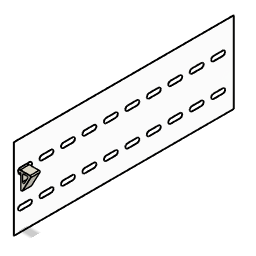
250711 TnH climate chamber wall shelf mount (Autodesk Fusion 360 design; units mm, degrees)
Autodesk Fusion 360 part; units mm, degrees
sketch "Sketch1" plane through (0, 0, 0) normal (1, 0, 0) x (0, 0, -1)
  line L0 (0, 0) -> (130.389561, 0) construction
  line L1 (0, 5) -> (20, 5)
  line L2 (0, -5) -> (20, -5)
  arc A0 (20, -5) -> (20, 5) centre (20, 0) ccw
  arc A1 (0, 5) -> (0, -5) centre (0, 0) ccw
  dimension "d1" = 10
  dimension "d2" = 10
  dimension "d3" = 20
  constraint coincident L0.start A1.centre
  constraint horizontal L0
  constraint coincident L0 A0.centre
  constraint tangent L1 A0
  constraint parallel L0 L1
  constraint tangent L2 A0
  constraint parallel L0 L2
  measures "d1" diameter of A0
  measures "d2" diameter of A1
  measures "d3" distance of L0.start A0.centre
extrude "Extrude1" add sketch "Sketch1" along normal blind 5 contours L1 L2 A0 A1 picked at (13.333333, -1.666667) makes body 1
pattern_linear "R-Pattern1" count 2 spacing 70 along (0, 1, 0) count 10 spacing 46 along (0, 0, -1) of bodies 1 makes body 2 at (0, 68.333333, -13.333333) makes body 3 at (0, -1.666667, -59.333333) makes body 4 at (0, 68.333333, -59.333333) makes body 5 at (0, -1.666667, -105.333333) makes body 6 at (0, 68.333333, -105.333333) makes body 7 at (0, -1.666667, -151.333333) makes body 8 at (0, 68.333333, -144.666667) makes body 9 at (0, -1.666667, -197.333333) makes body 10 at (0, 68.333333, -190.666667) makes body 11 at (0, -1.666667, -243.333333) makes body 12 at (0, 68.333333, -236.666667) makes body 13 at (0, -1.666667, -289.333333) makes body 14 at (0, 68.333333, -282.666667) makes body 15 at (0, -1.666667, -335.333333) makes body 16 at (0, 68.333333, -328.666667) makes body 17 at (0, -1.666667, -381.333333) makes body 18 at (0, 68.333333, -374.666667) makes body 19 at (0, -1.666667, -427.333333) makes body 20 at (0, 68.333333, -420.666667)
sketch "Sketch2" plane through (0, 0, 0) normal (1, 0, 0) x (0, 0, -1)
  line L0 (-13.995668, 128.760149) -> (457.458416, 128.760149)
  line L1 (457.458416, 128.760149) -> (457.458416, -45.186015)
  line L2 (457.458416, -45.186015) -> (-13.995668, -45.186015)
  line L3 (-13.995668, -45.186015) -> (-13.995668, 128.760149)
  constraint horizontal L0
  constraint vertical L1
  constraint horizontal L2
  constraint vertical L3
extrude "Extrude2" add sketch "Sketch2" along normal blind 1.1 separate body contours L0 L1 L2 L3 picked at (143.155693, 70.778094) makes body 21
combine "Combine1" operation cut target body 21 tool bodies 1 11 10 4 15 16 17 7 5 6 14 13 12 18 20 19 3 2 9 8 keep tools
ref_plane "WorkPlane1" through (-0.5, 0, -20) normal (0, 1, 0) x (-1, 0, 0)
sketch "Sketch3" plane through (0, 0, 0) normal (0, 1, 0) x (1, 0, 0)
  line L0 (-0.5, 20) -> (1.5, 20)
  line L1 (-0.5, 0) -> (1.5, 0)
  line L2 (0.5, 0) -> (0.5, 20)
  line L3 (0.5, 10, 0) -> (0.5, 10, 2.871027)
  line L4 (0.5, 10) -> (3.896403, 10)
  constraint midpoint L1 L2.start
  constraint midpoint L0 L2.end
  constraint midpoint L2 L4.start
  constraint perpendicular L2 L4
ref_plane "WorkPlane2" through (0.5, 0, -10) normal (0, 0, 1) x (1, 0, 0)
sketch "Sketch4" plane through (0, 0, -10) normal (0, 0, 1) x (1, 0, 0)
  line L0 (-4, 70) -> (21.1, 70)
  line L1 (0, 65) -> (0, 60.3)
  line L2 (0, 60.3) -> (-4, 60.3)
  line L3 (-4, 60.3) -> (-4, 70)
  line L4 (0, 65) -> (1.1, 65)
  line L5 (1.1, 65) -> (1.1, 34.146924)
  line L6 (22.865895, 67.061057) -> (4.865895, 33.20798)
  line L7 (7.1, 66) -> (14.442882, 66)
  line L8 (16.208777, 63.061057) -> (8.865895, 49.251104)
  line L9 (5.1, 50.190047) -> (5.1, 64)
  line L10 (0, 75) -> (1.1, 75) construction
  line L11 (1.1, 75) -> (1.1, 65) construction
  line L12 (1.1, 65) -> (0, 65) construction
  line L13 (0, 65) -> (0, 75) construction
  arc A0 (22.865895, 67.061057) -> (21.1, 70) centre (21.1, 68) ccw
  arc A1 (1.1, 34.146924) -> (4.865895, 33.20798) centre (3.1, 34.146924) ccw
  arc A2 (16.208777, 63.061057) -> (14.442882, 66) centre (14.442882, 64) ccw
  arc A3 (5.1, 50.190047) -> (8.865895, 49.251104) centre (7.1, 50.190047) ccw
  arc A4 (7.1, 66) -> (5.1, 64) centre (7.1, 64) ccw
  point P0 (1.1, -5)
  point P1 (1.1, 5)
  point P2 (0, 5)
  point P3 (0, -5)
  point P4 (1.1, 75)
  point P5 (1.1, 65)
  point P6 (0, 65)
  point P7 (0, 75)
  dimension "d12" = 9.7
  dimension "d13" = 4
  dimension "d14" = 5
  dimension "d15" = 4
  dimension "d16" = 4
  dimension "d17" = 4
  dimension "d18" = 2
  dimension "d19" = 2
  dimension "d20" = 62
  dimension "d21" = 20
  constraint horizontal L0
  constraint vertical L1
  constraint horizontal L2
  constraint vertical L3
  constraint perpendicular L1 L4
  constraint perpendicular L4 L5
  constraint perpendicular L5 L7
  constraint perpendicular L7 L9
  constraint coincident P5 L5
  constraint coincident P6 L1
  constraint horizontal L10
  constraint vertical L11
  constraint horizontal L12
  constraint vertical L13
  constraint coincident P5 L4.end
  constraint coincident P7 L10.start
  constraint collinear L4 L12
  constraint parallel L6 L8
  constraint tangent L0 A0
  constraint tangent L6 A0
  constraint tangent L5 A1
  constraint tangent L6 A1
  constraint equal A0 A1
  constraint tangent L7 A2
  constraint tangent L8 A2
  constraint tangent L8 A3
  constraint tangent L9 A3
  constraint equal A2 A3
  constraint tangent L7 A4
  constraint tangent L9 A4
  constraint equal A2 A4
  measures "d12" distance of L0 L2
  measures "d13" distance of L1 L3
  measures "d14" distance of L0 L4
  measures "d15" distance of L5 L9
  measures "d16" distance of L0 L7
  measures "d17" distance of L6 L8
  measures "d18" radius of A0
  measures "d19" radius of A2
  measures "d20" angle of L7 L8
  measures "d21" distance of L11 A0.centre
extrude "Extrude3" add sketch "Sketch4" along normal mid plane 20 separate body contours L0 L1 L2 L3 L4 L5 L6 A0 A1 picked at (12.199229, 49.840047) makes body 22
fillet "Fillet1" radius 1 2 edges at (-4, 60.3, -10) (0, 60.3, -10) on bodies 22
fillet "Fillet1" radius 4 1 edges at (-4, 70, -10) on bodies 22
fillet "Fillet2" radius 0.6 2 edges at (0, 65, -10) (1.1, 65, -10) on bodies 22
chamfer "Chamfer1" distance 0.4 angle 45 13 edges at (13.865895, 50.134519, -20) (22.814335, 69.030076, -20) (10.55, 70, -20) (-2.828427, 68.828427, -20) (-4, 63.65, -20) (-3.707107, 60.592893, -20) (-2, 60.3, -20) (-0.292893, 60.592893, -20) (0, 62.85, -20) (0.175736, 64.824264, -20) (0.954132, 64.792128, -20) (1.1, 49.277658, -20) (2.616156, 32.206332, -20) on bodies 22
fillet "Fillet3" radius 0.4 26 edges at (0.954132, 64.792128, -19.6) (1.1, 49.277658, -19.6) (2.616156, 32.206332, -19.6) (13.865895, 50.134519, -19.6) (22.814335, 69.030076, -19.6) (10.55, 70, -19.6) (-2.828427, 68.828427, -19.6) (-4, 63.65, -19.6) (-3.707107, 60.592893, -19.6) (-2, 60.3, -19.6) (-0.292893, 60.592893, -19.6) (0, 62.85, -19.6) (0.175736, 64.824264, -19.6) (22.814335, 69.030076, 0) (10.55, 70, 0) (-2.828427, 68.828427, 0) (-4, 63.65, 0) (-3.707107, 60.592893, 0) (-2, 60.3, 0) (-0.292893, 60.592893, 0) (0, 62.85, 0) (0.175736, 64.824264, 0) (13.865895, 50.134519, 0) (2.616156, 32.206332, 0) (1.1, 49.277658, 0) (0.954132, 64.792128, 0) on bodies 22
sketch "Sketch5" plane through (0, 0, -10) normal (0, 0, 1) x (1, 0, 0)
  line L0 (0, 5) -> (1.1, 5) construction
  line L1 (1.1, 5) -> (1.1, -5) construction
  line L2 (1.1, -5) -> (0, -5) construction
  line L3 (0, -5) -> (0, 5) construction
  line L4 (0, 75) -> (1.1, 75) construction
  line L5 (1.1, 75) -> (1.1, 65) construction
  line L6 (1.1, 65) -> (0, 65) construction
  line L7 (0, 65) -> (0, 75) construction
  line L8 (-3, 70) -> (21.1, 70)
  line L9 (0, 65) -> (0, 60.3)
  line L10 (0, 60.3) -> (-3, 60.3)
  line L11 (-3, 60.3) -> (-3, 70)
  line L12 (0, 65) -> (1.1, 65)
  line L13 (1.1, 65) -> (1.1, -1)
  line L14 (21.1, 70) -> (4.1, 51.119587)
  line L15 (4.1, 51.119587) -> (4.1, -8)
  line L16 (-3, -1) -> (1.1, -1)
  line L17 (0, -5) -> (0, -8)
  line L18 (0, -8) -> (-3, -8)
  line L19 (-3, -8) -> (-3, -1)
  line L20 (0, -5) -> (1.1, -5)
  line L21 (1.1, -5) -> (1.1, -8)
  line L22 (1.1, -8) -> (4.1, -8)
  line L23 (4.1, 67) -> (14.36189, 67)
  line L24 (14.36189, 67) -> (4.1, 55.603017)
  line L25 (4.1, 55.603017) -> (4.1, 67)
  point P0 (1.1, 75)
  point P1 (1.1, 65)
  point P2 (0, 65)
  point P3 (0, 75)
  point P4 (0, 5)
  point P5 (0, -5)
  point P6 (1.1, -5)
  point P7 (1.1, 5)
  dimension "d31" = 9.7
  dimension "d32" = 20
  dimension "d33" = 3
  dimension "d34" = 5
  dimension "d35" = 3
  dimension "d36" = 48
  dimension "d37" = 4
  dimension "d38" = 7
  dimension "d39" = 1.1
  dimension "d40" = 3
  dimension "d41" = 3
  dimension "d42" = 3
  dimension "d43" = 3
  constraint horizontal L0
  constraint vertical L1
  constraint horizontal L2
  constraint vertical L3
  constraint coincident P6 L1.end
  constraint coincident P4 L0.start
  constraint horizontal L4
  constraint vertical L5
  constraint horizontal L6
  constraint vertical L7
  constraint coincident P1 L5.end
  constraint coincident P3 L4.start
  constraint horizontal L8
  constraint vertical L9
  constraint horizontal L10
  constraint vertical L11
  constraint perpendicular L7 L12
  constraint collinear L7 L9
  constraint coincident L5 P1
  constraint perpendicular L12 L13
  constraint perpendicular L8 L15
  constraint horizontal L16
  constraint vertical L17
  constraint horizontal L18
  constraint vertical L19
  constraint perpendicular L3 L20
  constraint collinear L6 L12
  constraint collinear L2 L20
  constraint collinear L3 L17
  constraint perpendicular L18 L21
  constraint perpendicular L15 L22
  constraint collinear L18 L22
  constraint parallel L8 L23
  constraint parallel L14 L24
  constraint parallel L13 L25
  measures "d31" distance of L8 L10
  measures "d32" distance of L8.end L13
  measures "d33" distance of L9 L11
  measures "d34" distance of L8 L12
  measures "d35" distance of L17 L19
  measures "d36" angle of L8 L14
  measures "d37" distance of L16 L20
  measures "d38" distance of L16.start L18.end
  measures "d39" distance of L1 L3
  measures "d40" distance of L15 L21
  measures "d41" distance of L8 L23
  measures "d42" distance of L14 L24
  measures "d43" distance of L13 L25
extrude "Extrude4" add sketch "Sketch5" along normal mid plane 20 separate body contours L8 L9 L10 L11 L12 L13 L14 L15 L16 L17 L18 L19 L20 L21 L22 picked at (2.1, 38.373196) makes body 23
fillet "Fillet4" radius 1 1 edges at (21.1, 70, -10) on bodies 23
fillet "Fillet4" radius 3 1 edges at (4.1, 67, -10) on bodies 23
fillet "Fillet4" radius 1 1 edges at (14.36189, 67, -10) on bodies 23
fillet "Fillet4" radius 1 1 edges at (4.1, 55.603017, -10) on bodies 23
fillet "Fillet4" radius 57 1 edges at (4.1, 51.119587, -10) on bodies 23
fillet "Fillet5" radius 0.2 4 edges at (0, 65, -10) (1.1, 65, -10) (1.1, -5, -10) (0, -5, -10) on bodies 23
fillet "Fillet6" radius 1 6 edges at (-3, 60.3, -10) (0, 60.3, -10) (-3, 70, -10) (-3, -1, -10) (-3, -8, -10) (0, -8, -10) on bodies 23
fillet "Fillet6" radius 1 2 edges at (1.1, -8, -10) (4.1, -8, -10) on bodies 23
chamfer "Chamfer2" distance 3 distance2 2.5 1 edges at (1.1, -1, -10) measured on face at (1.1, 20.933333, -6.666667) on bodies 23
fillet "Fillet7" radius 10.5 2 edges at (-1.4, -1, -10) (1.1, 2, -10) on bodies 23
hidden bodies 23
named bodies: "steel panel", "single hole mount 62", "double hole mount"
